Shaft e1 v2 (Autodesk Fusion 360 design; units mm, degrees)
Autodesk Fusion 360 part; units mm, degrees
sketch "Sketch1" plane through (0, 0, 0) normal (0, 0, 1) x (1, 0, 0) in component "Shifted"
  circle A0 centre (-68.3204, 71.3613) radius 12.5
  circle A1 centre (0, 0) radius 8 construction
  circle A2 centre (0, 0) radius 6
  line L0 (0, 0) -> (0, 12.5) construction
  circle A3 centre (0, 8) radius 1.75
  circle A4 centre (-7.6085, 2.4721) radius 1.75
  circle A5 centre (-4.7023, -6.4721) radius 1.75
  circle A6 centre (4.7023, -6.4721) radius 1.75
  circle A7 centre (7.6085, 2.4721) radius 1.75
  circle A8 centre (0, 1) radius 12.4
  circle A9 centre (0, 1) radius 13.9
  dimension "d2" = 25
  dimension "d3" = 12
  dimension "d4" = 3.5
  dimension "d6" = 360
  dimension "d7" = 16
  dimension "d14" = 24.8
  dimension "d15" = 1
  dimension "d24" = 1.5
  constraint coincident A1.centre A2.centre
  constraint vertical L0
  constraint coincident A1 A3.centre
  constraint coincident L0 A3.centre
  constraint coincident L0 A8.centre
  measures "d2" diameter of A0
  measures "d3" diameter of A2
  measures "d4" diameter of A3
  measures "d7" diameter of A1
  measures "d14" diameter of A8
  measures "d15" distance of A1.centre A8.centre
extrude "Extrude1" add sketch "Sketch1" along normal blind 7 contours A8 makes body 1 in component "Shifted"
sketch "Sketch1 (2)" plane through (0, 0, 0) normal (0, 0, 1) x (1, 0, 0) in component "Normal"
  circle A0 centre (0, 0) radius 12.4
  circle A1 centre (0, 0) radius 8 construction
  circle A2 centre (0, 8) radius 1.75
  line L0 (0, 0) -> (0, 12.4) construction
  circle A3 centre (0, 0) radius 6
  circle A4 centre (-7.6085, 2.4721) radius 1.75
  circle A5 centre (-4.7023, -6.4721) radius 1.75
  circle A6 centre (4.7023, -6.4721) radius 1.75
  circle A7 centre (7.6085, 2.4721) radius 1.75
  circle A8 centre (0, 0) radius 13.9
  dimension "d16" = 24.8
  dimension "d17" = 16
  dimension "d18" = 3.5
  dimension "d19" = 12
  dimension "d21" = 360
  dimension "d27" = 1.5
  constraint coincident A0.centre A1.centre
  constraint coincident A1 A2.centre
  constraint coincident A0 L0.end
  constraint vertical L0
  constraint concentric A1 A3
  measures "d16" diameter of A0
  measures "d17" diameter of A1
  measures "d18" diameter of A2
  measures "d19" diameter of A3
extrude "Extrude1'" add sketch "Sketch1 (2)" along normal blind 7 separate body contours A0 makes body 2 in component "Normal"
extrude "Extrude1''" add sketch "Sketch1" against normal blind 2 contours A8 | A9 bodies 1 in component "Shifted"
extrude "Extrude2" add sketch "Sketch1 (2)" against normal blind 2 contours A0 | A8 bodies 2 in component "Normal"
sketch "Sketch1 (3)" plane through (0, 0, -2) normal (0, 0, -1) x (1, 0, 0) in component "Shifted2"
  circle A0 centre (0, 0) radius 6
  circle A1 centre (0, -8) radius 1.75
  circle A2 centre (-7.6085, -2.4721) radius 1.75
  circle A3 centre (-4.7023, 6.4721) radius 1.75
  circle A4 centre (7.6085, -2.4721) radius 1.75
  circle A5 centre (4.7023, 6.4721) radius 1.75
  circle A6 centre (0, -1) radius 13.9
  circle A7 centre (0, 0) radius 8 construction
  circle A8 centre (0, -8) radius 1.75
  circle A9 centre (7.6085, -2.4721) radius 1.75
  circle A10 centre (4.7023, 6.4721) radius 1.75
  circle A11 centre (-4.7023, 6.4721) radius 1.75
  circle A12 centre (-7.6085, -2.4721) radius 1.75
  line L0 (0, 0) -> (0, 8) construction
  circle A13 centre (0, 1) radius 12.4
  dimension "d30" = 16
  dimension "d31" = 3.5
  dimension "d33" = 360
  dimension "d35" = 24.8
  dimension "d37" = 1
  constraint concentric A0 A7
  constraint concentric A1 A8
  constraint coincident A0.centre A7.centre
  constraint coincident A7 L0.end
  constraint vertical L0
  measures "d30" diameter of A7
  measures "d31" diameter of A8
  measures "d35" diameter of A13
  measures "d37" distance of A0.centre A13.centre
extrude "Extrude3" add sketch "Sketch1 (3)" along normal blind 7 separate body contours A6 A13 | A6 A13 picked at (-8.0006, 3.6247) picked at (2.2451, 12.8454) makes body 3 in component "Shifted2"
sketch "Sketch2" plane through (0, 0, -9) normal (0, 0, -1) x (1, 0, 0) in component "Shifted2"
  circle A0 centre (7.6085, -2.4721) radius 1.75
  circle A1 centre (-7.6085, -2.4721) radius 1.75
  circle A2 centre (4.7023, 6.4721) radius 1.75
  circle A3 centre (0, -8) radius 1.75
  circle A4 centre (0, 0) radius 6
  circle A5 centre (-4.7023, 6.4721) radius 1.75
  circle A6 centre (0, 1) radius 12.4
  circle A7 centre (0, 1) radius 13.9
  dimension "d44" = 1.5
extrude "Extrude4" add sketch "Sketch2" along normal blind 2 contours A6 | A7 bodies 3 in component "Shifted2"
sketch "Sketch1 (4)" plane through (0, 0, 0) normal (0, 0, 1) x (1, 0, 0) in component "Normal (1)"
  circle A0 centre (0, 0) radius 12.4
  circle A1 centre (0, 0) radius 8 construction
  circle A2 centre (0, 8) radius 1.75
  line L0 (0, 0) -> (0, 12.4) construction
  circle A3 centre (0, 0) radius 6
  circle A4 centre (-7.6085, 2.4721) radius 1.75
  circle A5 centre (-4.7023, -6.4721) radius 1.75
  circle A6 centre (4.7023, -6.4721) radius 1.75
  circle A7 centre (7.6085, 2.4721) radius 1.75
  circle A8 centre (0, 0) radius 13.9
  dimension "d16_1" = 24.8
  dimension "d17_1" = 16
  dimension "d18_1" = 3.5
  dimension "d19_1" = 12
  dimension "d21_1" = 360
  dimension "d27_1" = 1.5
  constraint coincident A0.centre A1.centre
  constraint coincident A1 A2.centre
  constraint coincident A0 L0.end
  constraint vertical L0
  constraint concentric A1 A3
  measures "d16_1" diameter of A0
  measures "d17_1" diameter of A1
  measures "d18_1" diameter of A2
  measures "d19_1" diameter of A3
extrude "Extrude1'''" add sketch "Sketch1 (4)" along normal blind 7 separate body contours A0 makes body 4 in component "Normal (1)"
sketch "Sketch2 (2)" plane through (0, 0, -2) normal (0, 0, -1) x (1, 0, 0) in component "Normal"
  circle A0 centre (7.6085, -2.4721) radius 1.75
  circle A1 centre (4.7023, 6.4721) radius 1.75
  circle A2 centre (-4.7023, 6.4721) radius 1.75
  circle A3 centre (-7.6085, -2.4721) radius 1.75
  circle A4 centre (0, 0) radius 6
  circle A5 centre (0, -8) radius 1.75
  circle A6 centre (0, 0) radius 13.9
  circle A7 centre (0, -1) radius 12.4
  circle A8 centre (0, -1) radius 13.9
  dimension "d51" = 1.5
extrude "Extrude3'" add sketch "Sketch2 (2)" along normal blind 2 contours A6 A8 | A6 A8 | A7 picked at (-13.2742, 0.622) picked at (-0.0833, -14.2078) bodies 2 in component "Normal"
sketch "Sketch1 (1)" plane through (0, 0, -2) normal (0, 0, -1) x (1, 0, 0) in component "Shifted"
  circle A0 centre (0, 0) radius 6
  circle A1 centre (0, -8) radius 1.75
  circle A2 centre (-7.6085, -2.4721) radius 1.75
  circle A3 centre (-4.7023, 6.4721) radius 1.75
  circle A4 centre (7.6085, -2.4721) radius 1.75
  circle A5 centre (4.7023, 6.4721) radius 1.75
  circle A6 centre (0, -1) radius 13.9
  circle A7 centre (0, 1) radius 12.4
  circle A8 centre (0, 1) radius 12.4
  circle A9 centre (0, 1) radius 13.9
  dimension "d54" = 1.5
extrude "Extrude2'" add sketch "Sketch1 (1)" along normal blind 2 contours A6 A7 A8 A9 | A6 A7 A8 A9 | A6 A7 A8 | A6 A7 A8 bodies 1 in component "Shifted"
sketch "Sketch3" plane through (0, 0, -11) normal (0, 0, -1) x (1, 0, 0) in component "Shifted2"
  circle A0 centre (7.6085, -2.4721) radius 1.75
  circle A1 centre (-7.6085, -2.4721) radius 1.75
  circle A2 centre (0, -8) radius 1.75
  circle A3 centre (4.7023, 6.4721) radius 1.75
  circle A4 centre (-4.7023, 6.4721) radius 1.75
  circle A5 centre (0, 0) radius 6
  circle A6 centre (0, 1) radius 13.9
  circle A7 centre (0, 0) radius 12.4
  circle A8 centre (0, 0) radius 12.4
  circle A9 centre (0, 0) radius 13.9
  dimension "d57" = 1.5
extrude "Extrude5" add sketch "Sketch3" along normal blind 2 contours A6 A9 | A6 A9 | A7 A8 picked at (-13.2742, 1.622) picked at (-0.0833, -13.2078) bodies 3 in component "Shifted2"
component "Shifted" placed x (1, 0, 0) y (0, 1, 0) z (0, 0, 1) at (0, 0, -2)
component "Normal" placed x (1, 0, 0) y (0, 1, 0) z (0, 0, 1) at (0, 0, 9)
component "Shifted2" placed x (1, 0, 0) y (0, 1, 0) z (0, 0, 1) at (0, 0, -4)
component "Normal (1)" placed x (1, 0, 0) y (0, 1, 0) z (0, 0, 1) at (0, 0, -24)
